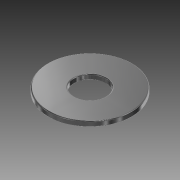
# Autodesk Inventor part: Washer(M3)
Saved by Autodesk Inventor 2013 (Build 170138000, 138)
## iProperties
Created: 2012-10-26
Material: ステンレス鋼
Document SubType Name: Modeling
Designer: andou
Density: 8.08 g/cm^3
Mass: 0.173317 g
Surface Area: 1.00706 cm^2
Volume: 0.0214501 cm^3
Author: andou
Title: Washer(M3)
Autodesk Inventor part; units mm, degrees
ref_plane "YZ Plane" through (0, 0, 0) normal (1, 0, 0) x (0, 1, 0)
ref_plane "XZ Plane" through (0, 0, 0) normal (0, 1, 0) x (-1, 0, 0)
ref_plane "XY Plane" through (0, 0, 0) normal (0, 0, 1) x (1, 0, 0)
sketch "スケッチ1" plane through (0, 0, 0) normal (0, 0, 1) x (1, 0, 0)
  circle A0 centre (0, 0) radius 4
  circle A1 centre (0, 0) radius 1.5
  dimension "d0" = 8
  dimension "d1" = 3
  constraints: 2 centre point, 2 coincident
  measures "d0" diameter of A0
  measures "d1" diameter of A1
extrude "押し出し1" add sketch "スケッチ1" along normal blind 0.5
fillet "フィレット1" radius 0.1 4 edges at (-4, 0, 0.5) (-1.5, 0, 0.5) (-4, 0, 0) (-1.5, 0, 0)
